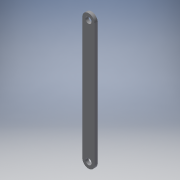
# Autodesk Inventor part: part2
Saved by Autodesk Inventor 2016 (Build 200138000, 138)
## iProperties
Created: 2017-09-07
Part Number: part2
Material: Generic
Document SubType Name: Modeling
Designer: student
Density: 1 g/cm^3
Appearance: Default
Author: student
Autodesk Inventor part; units mm, degrees
ref_plane "YZ Plane" through (0, 0, 0) normal (1, 0, 0) x (0, 1, 0)
ref_plane "XZ Plane" through (0, 0, 0) normal (0, 1, 0) x (-1, 0, 0)
ref_plane "XY Plane" through (0, 0, 0) normal (0, 0, 1) x (1, 0, 0)
sketch "Sketch1" plane through (0, 0, 0) normal (0, 0, 1) x (1, 0, 0)
  line L0 (-23.739, 2.1473) -> (-23.739, 129.1473) construction
  line L1 (-17.389, 2.1473) -> (-17.389, 129.1473)
  line L2 (-30.089, 129.1473) -> (-30.089, 2.1473)
  arc A0 (-30.089, 2.1473) -> (-17.389, 2.1473) centre (-23.739, 2.1473) ccw
  arc A1 (-17.389, 129.1473) -> (-30.089, 129.1473) centre (-23.739, 129.1473) ccw
  circle A2 centre (-23.739, 129.1473) radius 3.175
  circle A3 centre (-23.739, 2.1473) radius 3.175
  circle A4 centre (0, 0) radius 3.175 construction
  point P0 (-23.739, 65.6473)
  dimension "d0" = 127
  dimension "d1" = 12.7
  dimension "d2" = 6.35
  dimension "d3" = 6.35
  dimension "d4" = 6.35
  constraints: 8 end point, 4 centre point, 4 point on circle, 4 tangent, 2 coincident, 1 midpoint, 1 parallel, 1 vertical
  measures "d0" distance of L0.start L0.end
  measures "d1" diameter of A1
  measures "d2" diameter of A4
  measures "d3" diameter of A3
  measures "d4" diameter of A2
extrude "Extrusion1" add sketch "Sketch1" along normal blind 3.175
equation "\"d3\" = d2"
equation "\"d4\" = d2"
body "Solid1"
